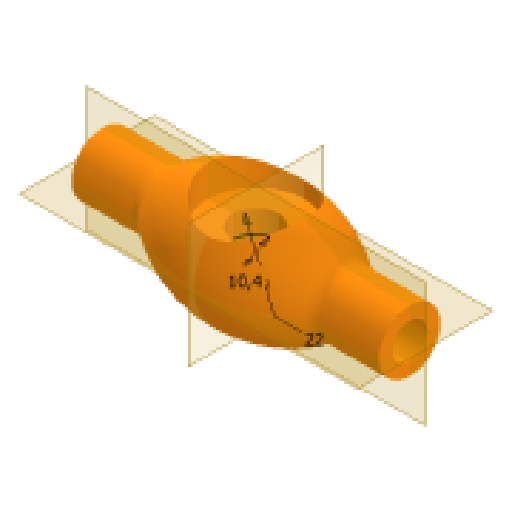
# Autodesk Inventor part: Крепление ходовой гайки
Saved by Autodesk Inventor 2023.2 (Build 272271030, 271C)
## iProperties
Created: 2025-04-02
Part Number: Крепление ходовой гайки
Material: Типовые
Document SubType Name: Modeling
Designer: Коноваленко
Density: 1 g/cm^3
Appearance: По умолчанию
Author: Коноваленко
Autodesk Inventor part; units mm, degrees
ref_plane "YZ Plane" through (0, 0, 0) normal (1, 0, 0) x (0, 1, 0)
ref_plane "XZ Plane" through (0, 0, 0) normal (0, 1, 0) x (-1, 0, 0)
ref_plane "XY Plane" through (0, 0, 0) normal (0, 0, 1) x (1, 0, 0)
sketch "Эскиз1" plane through (0, 0, 0) normal (0, 0, 1) x (1, 0, 0)
  line L0 (-35, 0) -> (-35, 7)
  line L1 (-35, 7) -> (0, 7)
  line L2 (-49, 0) -> (49, 0) projected
  line L3 (0, 20.2666) -> (0, -30.2111) projected
  line L4 (35, 0) -> (35, 7)
  line L5 (35, 7) -> (0, 7)
  arc A0 (20, 7) -> (-20, 7) centre (0, -23) ccw
  point P0 (0, 0)
  dimension "d0" = 7
  dimension "d1" = 35
  dimension "d4" = 40
  dimension "d5" = 30
  constraints: 8 end point, 5 point on line, 2 point on circle, 2 symmetric about line, 1 centre point, 1 perpendicular, 1 vertical
  measures "d0" distance of L0.start L0.end
  measures "d1" distance of L0.end L1.end
  measures "d4" distance of A0.end A0.start
  measures "d5" distance from line of L1 A0.centre
revolve "Вращение1" add sketch "Эскиз1" angle 360 about axis through (0, 0, 0) along (1, 0, 0)
fillet "Сопряжение1" radius 5 2 edges at (20, -7, 0) (-20, -7, 0)
sketch "Эскиз2" plane through (-35, 0, 0) normal (-1, 0, 0) x (0, 0, 1)
  circle A0 centre (0, 0) radius 4.1
  dimension "d7" = 8.2
  constraints: 1 centre point, 1 coincident
  measures "d7" diameter of A0
extrude "Выдавливание1" cut sketch "Эскиз2" against normal blind 17
sketch "Эскиз3" plane through (35, 0, 0) normal (1, 0, 0) x (0, 0, -1)
  circle A0 centre (0, 0) radius 4
  dimension "d10" = 8
  constraints: 1 centre point, 1 coincident
  measures "d10" diameter of A0
extrude "Выдавливание2" cut sketch "Эскиз3" against normal blind 17
sketch "Эскиз4" plane through (0, 0, 0) normal (0, 1, 0) x (-1, 0, 0)
  circle A0 centre (0, 0) radius 5.2
  circle A1 centre (0, 0) radius 11
  dimension "d13" = 10.4
  dimension "d16" = 22
  constraints: 2 centre point, 2 coincident
  measures "d13" diameter of A0
  measures "d16" diameter of A1
extrude "Выдавливание3" cut sketch "Эскиз4" against normal blind 17 contours A0
extrude "Выдавливание4" cut sketch "Эскиз4" along normal blind 17 contours A0 | A1
sketch "Эскиз5" plane through (0, 0, 0) normal (0, 1, 0) x (1, 0, 0)
  circle A0 centre (0, 0) radius 5.2 projected
  circle A1 centre (0, 0) radius 11 projected
extrude "Выдавливание5" add sketch "Эскиз4" along normal blind 5
sketch "Эскиз6" plane through (0, 5, 0) normal (0, 1, 0) x (1, 0, 0)
  circle A0 centre (-8, 0) radius 1.75 projected
  circle A1 centre (0, -8) radius 1.75 projected
  circle A2 centre (8, 0) radius 1.75 projected
  circle A3 centre (0, 8) radius 1.75 projected
  point P0 (0, 0)
extrude "Выдавливание6" cut sketch "Эскиз6" against normal blind 5
